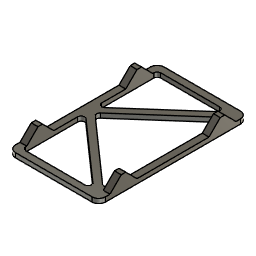
battery shim v4 (Autodesk Fusion 360 design; units mm, degrees)
Autodesk Fusion 360 part; units mm, degrees
sketch "Sketch1" plane through (0, 0, 0) normal (0, 0, 1) x (1, 0, 0)
  line L0 (0, 0) -> (40, 0)
  line L1 (40, 0) -> (40, 66)
  line L2 (40, 66) -> (0, 66)
  line L3 (0, 66) -> (0, 0)
  line L4 (3, 3) -> (37, 3)
  line L5 (37, 3) -> (37, 63)
  line L6 (37, 63) -> (3, 63)
  line L7 (3, 63) -> (3, 3)
  dimension "d3" = 66
  dimension "d4" = 40
  dimension "d7" = -3
  constraint horizontal L0
  constraint vertical L1
  constraint horizontal L2
  constraint vertical L3
  constraint coincident L0.start L3.end
  measures "d3" distance of L0.start L2.end
  measures "d4" distance of L0.start L0.end
extrude "Extrude1" add sketch "Sketch1" along normal blind 2
sketch "Sketch2" plane through (0, 0, 0) normal (1, 0, 0) x (0, 1, 0)
  line L0 (61, 2) -> (56, 7)
  line L1 (56, 7) -> (54, 7)
  line L2 (54, 7) -> (49, 2)
  line L3 (49, 2) -> (61, 2)
  line L4 (66, 2) -> (0, 2) construction
  line L5 (33, 2) -> (33, 19) construction
  line L6 (5, 2) -> (10, 7)
  line L7 (10, 7) -> (12, 7)
  line L8 (12, 7) -> (17, 2)
  line L9 (17, 2) -> (5, 2)
  dimension "d10" = 5
  dimension "d11" = 45
  dimension "d12" = 2
  dimension "d13" = 5
  constraint horizontal L1
  constraint parallel L1 L3
  constraint midpoint L4 L5.start
  constraint perpendicular L4 L5
  constraint coincident L2.end L4
  constraint equal L0 L2
  constraint symmetric L0.start L5 L6.start
  constraint symmetric L0.end L5 L6.end
  constraint symmetric L1.end L5 L7.end
  constraint symmetric L2.end L5 L8.end
  measures "d10" distance of L1 L3
  measures "d11" angle of L0 L3
  measures "d12" distance of L0.end L1.end
  measures "d13" distance of L0.start L4.start
extrude "Extrude2" add sketch "Sketch2" along normal up to surface (3 mm away)
extrude "Extrude3" add sketch "Sketch2" along normal up to surface (3 mm away) from surface at 37
sketch "Sketch3" plane through (0, 0, 2) normal (0, 0, 1) x (-1, 0, 0)
  line L0 (0, -17) -> (-3, -17)
  line L1 (-3, -17) -> (-3, -49)
  line L2 (-3, -49) -> (0, -49)
  line L3 (0, -49) -> (0, -17)
  line L4 (-37, -63) -> (-3, -33) construction
  line L5 (-3, -33) -> (-37, -3) construction
  line L6 (-36.0076, -64.1248) -> (-0.7328, -33)
  line L7 (-0.7328, -33) -> (-36.0076, -1.8752)
  line L8 (-37.9924, -61.8752) -> (-5.2672, -33)
  line L9 (-5.2672, -33) -> (-37.9924, -4.1248)
  line L10 (-37, -63) -> (-34.7328, -63)
  line L11 (-37, -63) -> (-37, -60.9996)
  line L12 (-37, -3) -> (-37, -5.0004)
  line L13 (-37, -3) -> (-34.7328, -3)
  line L14 (-3, -30.9996) -> (-3, -35.0004)
  point P0 (-37, -3)
  point P1 (-37, -63)
  dimension "d19" = 1.5
  dimension "d20" = -1.5
  constraint midpoint L1 L4.end
  constraint coincident P0 L5.end
  constraint coincident P1 L4.start
  constraint coincident L6 L10.end
  constraint horizontal L10
  constraint coincident L8 L11.end
  constraint perpendicular L10 L11
  constraint coincident L9 L12.end
  constraint parallel L11 L12
  constraint coincident L7 L13.end
  constraint perpendicular L12 L13
  constraint coincident L7 L14.start
  constraint coincident L1 L14.start
  constraint coincident L6 L14.end
  constraint coincident L1 L14.end
extrude "Extrude4" add sketch "Sketch3" against normal up to surface (2 mm away) contours L1 L6 L7 L8 L9 L10 L11 L12 L13 L14
fillet "Fillet1" radius 1.5 9 edges at (3, 63, 1) (3, 35.0004, 1) (3, 30.9996, 1) (34.7328, 63, 1) (37, 60.9996, 1) (37, 5.0004, 1) (34.7328, 3, 1) (3, 3, 1) (5.2672, 33, 1)
fillet "Fillet2" radius 3 4 edges at (40, 0, 1) (40, 66, 1) (0, 66, 1) (0, 0, 1)
equation "encl_depth = 66 mm"
equation "shim_H = 5 mm"
equation "d3 = encl_depth"
equation "wall_t = 2 mm"
equation "clearance = 0.2 mm"
equation "d8 = wall_t"
equation "d10 = shim_H"
